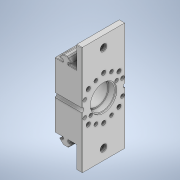
# Autodesk Inventor part: BearingMount
Saved by Autodesk Inventor 2020 (Build 240168000, 168)
## iProperties
Created: 2020-01-07
Part Number: BearingMount
Material: Generic
Document SubType Name: Modeling
Designer: srini
Density: 1 g/cm^3
Appearance: Default
Author: srini
Autodesk Inventor part; units mm, degrees
ref_plane "YZ Plane" through (0, 0, 0) normal (1, 0, 0) x (0, 1, 0)
ref_plane "XZ Plane" through (0, 0, 0) normal (0, 1, 0) x (-1, 0, 0)
ref_plane "XY Plane" through (0, 0, 0) normal (0, 0, 1) x (1, 0, 0)
sketch "Sketch1" plane through (0, 0, 0) normal (0, 0, 1) x (1, 0, 0)
  arc A0 (3.4842, -10.3402) -> (2.8892, -12.7) centre (3.4842, -11.5951) ccw construction
  line L0 (3.4842, -10.3402) -> (5.6567, -10.3402) construction
  arc A1 (5.6567, -10.3402) -> (6.269, -8.8618) centre (5.6567, -9.4742) ccw construction
  line L1 (6.269, -8.8618) -> (2.9517, -5.5445) construction
  line L2 (0.8127, -4.6585) -> (-2.4489, -4.6585) construction
  arc A2 (2.9517, -5.5445) -> (0.8127, -4.6585) centre (0.8127, -7.6835) ccw construction
  arc A3 (-2.4489, -4.6585) -> (-4.5879, -5.5445) centre (-2.4489, -7.6835) ccw construction
  line L3 (-4.5879, -5.5445) -> (-7.9053, -8.8618) construction
  arc A4 (-7.9053, -8.8618) -> (-7.2929, -10.3402) centre (-7.2929, -9.4742) ccw construction
  line L4 (-7.2929, -10.3402) -> (-5.1204, -10.3402) construction
  arc A5 (-4.5255, -12.7) -> (-5.1204, -10.3402) centre (-5.1204, -11.5951) ccw construction
  arc A6 (2.8892, -88.9) -> (3.4842, -91.2598) centre (3.4842, -90.0049) ccw construction
  line L5 (5.6567, -91.2598) -> (3.4842, -91.2598) construction
  arc A7 (6.269, -92.7382) -> (5.6567, -91.2598) centre (5.6567, -92.1258) ccw construction
  line L6 (2.9517, -96.0555) -> (6.269, -92.7382) construction
  arc A8 (0.8127, -96.9415) -> (2.9517, -96.0555) centre (0.8127, -93.9165) ccw construction
  line L7 (-2.4489, -96.9415) -> (0.8127, -96.9415) construction
  arc A9 (-4.5879, -96.0555) -> (-2.4489, -96.9415) centre (-2.4489, -93.9165) ccw construction
  line L8 (-7.9053, -92.7382) -> (-4.5879, -96.0555) construction
  arc A10 (-7.2929, -91.2598) -> (-7.9053, -92.7382) centre (-7.2929, -92.1258) ccw construction
  line L9 (-5.1204, -91.2598) -> (-7.2929, -91.2598) construction
  arc A11 (-5.1204, -91.2598) -> (-4.5255, -88.9) centre (-5.1204, -90.0049) ccw construction
  line L10 (18.2319, -12.7) -> (2.8892, -12.7)
  line L11 (-13.5181, -12.7) -> (-13.5181, -88.9)
  line L12 (-13.5181, -88.9) -> (-4.5255, -88.9)
  line L13 (18.2319, -88.9) -> (18.2319, -12.7)
  line L14 (-13.5181, -6.3246) -> (-13.5181, -9.5504) projected
  line L15 (2.8892, -12.7) -> (2.4625, -12.7)
  line L16 (-4.5255, -12.7) -> (-13.5181, -12.7)
  line L17 (2.8892, -88.9) -> (18.2319, -88.9)
  line L18 (-4.5255, -88.9) -> (-4.0987, -88.9)
  line L19 (18.2319, 12.7) -> (11.8819, 12.7)
  line L20 (11.8819, 12.7) -> (11.8819, -114.3)
  line L21 (11.8819, -114.3) -> (18.2319, -114.3)
  line L22 (18.2319, -114.3) -> (18.2319, 12.7)
  line L23 (8.7323, 12.7) -> (5.5065, 12.7) projected
  arc A12 (2.4625, -88.9) -> (3.4842, -91.5098) centre (3.4842, -90.0049) ccw
  line L24 (3.4842, -91.5098) -> (5.6567, -91.5098)
  arc A13 (6.0922, -92.5614) -> (5.6567, -91.5098) centre (5.6567, -92.1258) ccw
  line L25 (6.0922, -92.5614) -> (2.7749, -95.8787)
  arc A14 (0.8127, -96.6915) -> (2.7749, -95.8787) centre (0.8127, -93.9165) ccw
  line L26 (0.8127, -96.6915) -> (-2.4489, -96.6915)
  arc A15 (-4.4112, -95.8787) -> (-2.4489, -96.6915) centre (-2.4489, -93.9165) ccw
  line L27 (-4.4112, -95.8787) -> (-7.7285, -92.5614)
  arc A16 (-7.2929, -91.5098) -> (-7.7285, -92.5614) centre (-7.2929, -92.1258) ccw
  line L28 (-7.2929, -91.5098) -> (-5.1204, -91.5098)
  arc A17 (-5.1204, -91.5098) -> (-4.0987, -88.9) centre (-5.1204, -90.0049) ccw
  line L29 (-4.0987, -88.9) -> (2.4625, -88.9)
  line L30 (2.4625, -88.9) -> (2.8892, -88.9)
  arc A18 (-4.0987, -12.7) -> (-5.1204, -10.0902) centre (-5.1204, -11.5951) ccw
  line L31 (-5.1204, -10.0902) -> (-7.2929, -10.0902)
  arc A19 (-7.7285, -9.0386) -> (-7.2929, -10.0902) centre (-7.2929, -9.4742) ccw
  line L32 (-7.7285, -9.0386) -> (-4.4112, -5.7213)
  arc A20 (-2.4489, -4.9085) -> (-4.4112, -5.7213) centre (-2.4489, -7.6835) ccw
  line L33 (-2.4489, -4.9085) -> (0.8127, -4.9085)
  arc A21 (2.7749, -5.7213) -> (0.8127, -4.9085) centre (0.8127, -7.6835) ccw
  line L34 (2.7749, -5.7213) -> (6.0922, -9.0386)
  arc A22 (5.6567, -10.0902) -> (6.0922, -9.0386) centre (5.6567, -9.4742) ccw
  line L35 (5.6567, -10.0902) -> (3.4842, -10.0902)
  arc A23 (3.4842, -10.0902) -> (2.4625, -12.7) centre (3.4842, -11.5951) ccw
  line L36 (-4.0987, -12.7) -> (-4.5255, -12.7)
  line L37 (2.4625, -12.7) -> (-4.0987, -12.7)
  point P0 (0, 0)
  point P1 (11.8819, -12.7)
  point P2 (11.8819, -88.9)
  dimension "d0" = 31.75
  dimension "d1" = 127
  dimension "d2" = 6.35
  dimension "d81" = 0.25
  dimension "d82" = 0.25
  constraints: 52 end point, 28 parallel, 28 point on circle, 12 centre point, 6 horizontal, 6 perpendicular, 3 collinear, 1 point on line, 20 other
  measures "d0" distance of L10.start L11.start
  measures "d1" distance of L21.end L19.start
  measures "d2" distance of L19.start L19.end
  measures "d81" distance between parallel lines of L26 L7
  measures "d82" distance between parallel lines of L2 L33
extrude "Extrusion1" add sketch "Sketch1" along normal blind 50.8
sketch "Sketch2" plane through (18.2319, -114.3, 0) normal (1, 0, 0) x (0, 0, -1)
  circle A0 centre (-12.7, 114.3) radius 3.3734
  line L0 (0, 127) -> (-50.8, 127) projected
  line L1 (0, 0) -> (0, 127) projected
  circle A1 centre (-12.7, 12.7) radius 3.3734
  circle A2 centre (-25.4, 114.3) radius 3.3734
  circle A3 centre (-25.4, 12.7) radius 3.3734
  circle A4 centre (-25.4, 63.5) radius 12.9921
  circle A5 centre (-38.1, 114.3) radius 3.3734
  circle A6 centre (-38.1, 12.7) radius 3.3734
  point P0 (0, 114.3)
  dimension "d5" = 12.7
  dimension "d6" = 12.7
  dimension "d7" = 6.7469
  dimension "d10" = 101.6
  dimension "d13" = 12.7
  dimension "d29" = 63.5
  dimension "d30" = 25.4
  dimension "d31" = 25.9842
  constraints: 7 centre point, 1 horizontal, 1 vertical, 10 other
  measures "d5" distance from line of A0.centre L0
  measures "d6" distance from line of A0.centre L1
  measures "d7" diameter of A0
  measures "d10" distance of A0.centre A1.centre
  measures "d13" distance of A0.centre A2.centre
  measures "d29" distance from line of A4.centre L0
  measures "d30" distance from line of A4.centre L1
  measures "d31" diameter of A4
extrude "Extrusion2" cut sketch "Sketch2" against normal through all contours A2 | A3 | A4
sketch "Sketch4" plane through (18.2319, -114.3, 0) normal (1, 0, 0) x (0, 0, -1)
  circle A0 centre (-25.4, 63.5) radius 12.9921 projected
  circle A1 centre (-25.4, 63.5) radius 14.3002
  point P0 (0, 114.3)
  dimension "d32" = 28.6004
  constraints: 1 centre point, 1 coincident
  measures "d32" diameter of A1
extrude "Extrusion4" cut sketch "Sketch4" against normal blind 7.9756 contours A0 | A1
sketch "Sketch5" plane through (18.2319, -114.3, 0) normal (1, 0, 0) x (0, 0, -1)
  circle A0 centre (-25.4, 63.5) radius 14.3002 projected
  circle A1 centre (-25.4, 63.5) radius 15.5702
  point P0 (0, 114.3)
  dimension "d35" = 31.1404
  constraints: 1 centre point, 1 coincident
  measures "d35" diameter of A1
extrude "Extrusion5" cut sketch "Sketch5" against normal blind 1.6256 contours A0 | A1
sketch "Sketch6" plane through (-13.5181, -88.9, 0) normal (-1, 0, 0) x (0, 0, 1)
  circle A0 centre (25.4, 38.1) radius 12.9921 projected
  circle A1 centre (25.4, 38.1) radius 14.3002
  point P0 (0, 88.9)
  dimension "d41" = 28.6004
  constraints: 1 centre point, 1 coincident
  measures "d41" diameter of A1
extrude "Extrusion6" cut sketch "Sketch6" against normal blind 7.9756 contours A0 | A1
sketch "Sketch7" plane through (-13.5181, -88.9, 0) normal (-1, 0, 0) x (0, 0, 1)
  circle A0 centre (25.4, 38.1) radius 14.3002 projected
  circle A1 centre (25.4, 38.1) radius 15.5702
  point P0 (0, 88.9)
  dimension "d44" = 31.1404
  constraints: 1 centre point, 1 coincident
  measures "d44" diameter of A1
extrude "Extrusion7" cut sketch "Sketch7" against normal blind 1.6256 contours A0 | A1
sketch "Sketch8" plane through (-13.5181, -88.9, 0) normal (-1, 0, 0) x (0, 0, 1)
  circle A0 centre (10.3089, 48.1835) radius 2.0955
  circle A1 centre (40.4911, 28.0165) radius 2.0955
  line L0 (10.3089, 48.1835) -> (40.4911, 28.0165)
  circle A2 centre (25.4, 38.1) radius 12.9921 projected
  line L1 (50.8, -25.4) -> (50.8, 101.6) projected
  point P0 (0, 88.9)
  dimension "d50" = 36.2998
  dimension "d51" = 4.191
  dimension "d74" = 56.25
  constraints: 2 centre point, 2 end point, 1 coincident, 1 equal radius, 1 midpoint
  measures "d50" distance of L0.start L0.end
  measures "d51" diameter of A0
  measures "d74" angle of L0 L1
extrude "Extrusion8" cut sketch "Sketch8" against normal through all contours A0 | A1
chamfer "Chamfer3" distance 0.635 angle 45 18 edges at (11.8819, 0, 50.8) (-13.5181, -50.8, 50.8) (15.0569, 12.7, 50.8) (18.2319, -50.8, 50.8) (11.8819, -101.6, 50.8) (15.0569, -114.3, 50.8) (15.0569, -114.3, 0) (11.8819, -101.6, 0) (-13.5181, -50.8, 0) (18.2319, -50.8, 0) (11.8819, 0, 0) (15.0569, 12.7, 0) (11.8819, -101.6, 28.7734) (18.2319, -101.6, 28.7734) (18.2319, 0, 28.7734) (11.8819, 0, 28.7734) (-13.5181, -12.7, 25.4) (-13.5181, -88.9, 25.4)
sketch "Sketch9" plane through (18.2319, -114.3, 0.635) normal (1, 0, 0) x (0, 0, -1)
  circle A0 centre (-24.765, 38.1) radius 2.4892
  circle A1 centre (-24.765, 63.5) radius 12.9921 projected
  circle A2 centre (-6.8045, 45.5395) radius 2.4892
  circle A3 centre (0.635, 63.5) radius 2.4892
  circle A4 centre (-6.8045, 81.4605) radius 2.4892
  circle A5 centre (-24.765, 88.9) radius 2.4892
  circle A6 centre (-42.7255, 81.4605) radius 2.4892
  circle A7 centre (-50.165, 63.5) radius 2.4892
  circle A8 centre (-42.7255, 45.5395) radius 2.4892
  point P0 (0.635, 114.3)
  dimension "d57" = 25.4
  dimension "d58" = 4.9784
  dimension "d61" = 360
  constraints: 8 centre point, 1 vertical alignment, 17 other
  measures "d57" distance of A1.centre A0.centre
  measures "d58" diameter of A0
extrude "Extrusion9" cut sketch "Sketch9" against normal through all contours A0 | A2 | A3 | A4 | A5 | A6 | A7 | A8
sketch "Sketch10" plane through (-13.5181, -88.9, 0.635) normal (-1, 0, 0) x (0, 0, 1)
  circle A0 centre (15.6524, 16.1001) radius 2.1526
  circle A1 centre (24.765, 38.1) radius 12.9921 construction
  circle A2 centre (24.765, 12.7) radius 2.4892 projected
  line L0 (24.765, 12.7) -> (24.765, 38.1) construction
  line L1 (24.765, 38.1) -> (15.6524, 16.1001) construction
  line L2 (24.765, 38.1) -> (33.8776, 16.1001) construction
  circle A3 centre (33.8776, 16.1001) radius 2.1526
  line L3 (24.765, 38.1) -> (46.7649, 28.9874) construction
  circle A4 centre (46.7649, 28.9874) radius 2.1526
  line L4 (24.765, 38.1) -> (46.7649, 47.2126) construction
  circle A5 centre (46.7649, 47.2126) radius 2.1526
  line L5 (24.765, 38.1) -> (33.8776, 60.0999) construction
  circle A6 centre (33.8776, 60.0999) radius 2.1526
  line L6 (24.765, 38.1) -> (15.6524, 60.0999) construction
  circle A7 centre (15.6524, 60.0999) radius 2.1526
  line L7 (24.765, 38.1) -> (2.7651, 47.2126) construction
  circle A8 centre (2.7651, 47.2126) radius 2.1526
  line L8 (24.765, 38.1) -> (2.7651, 28.9874) construction
  circle A9 centre (2.7651, 28.9874) radius 2.1526
  point P0 (-0.635, 88.9)
  dimension "d65" = 4.3053
  dimension "d66" = 23.8125
  dimension "d67" = 22.5
  dimension "d70" = 360
  constraints: 18 end point, 8 centre point, 2 coincident, 1 vertical, 31 other
  measures "d65" diameter of A0
  measures "d66" distance of L0.end L1.end
  measures "d67" angle of L1 L0
extrude "Extrusion10" cut sketch "Sketch10" against normal through all contours A0 | A3 | A4 | A5 | A6 | A7 | A8 | A9
sketch "Sketch11" plane through (11.8819, -12.7, 0.635) normal (-1, 0, 0) x (0, 0, 1)
  line L0 (28.1384, 9.3266) -> (21.3916, 9.3266)
  line L1 (21.3916, 9.3266) -> (21.3916, 16.0734)
  line L2 (21.3916, 16.0734) -> (28.1384, 16.0734)
  line L3 (28.1384, 16.0734) -> (28.1384, 9.3266)
  circle A0 centre (24.765, 12.7) radius 3.3734 projected
  line L4 (28.1384, 9.3266) -> (21.3916, 16.0734) construction
  line L5 (21.3916, 9.3266) -> (28.1384, 16.0734) construction
  line L6 (28.1384, -85.5266) -> (21.3916, -85.5266)
  line L7 (21.3916, -85.5266) -> (21.3916, -92.2734)
  line L8 (21.3916, -92.2734) -> (28.1384, -92.2734)
  line L9 (28.1384, -92.2734) -> (28.1384, -85.5266)
  circle A1 centre (24.765, -88.9) radius 3.3734 projected
  line L10 (28.1384, -85.5266) -> (21.3916, -92.2734) construction
  line L11 (21.3916, -85.5266) -> (28.1384, -92.2734) construction
  point P0 (-0.635, 12.7)
  constraints: 24 end point, 4 midpoint, 4 parallel, 4 tangent, 2 horizontal, 2 perpendicular
extrude "Extrusion11" cut sketch "Sketch11" against normal blind 3.175
sketch "Sketch12" plane through (11.8819, -114.3, 0.635) normal (-1, 0, 0) x (0, 0, 1)
  circle A0 centre (24.765, 12.7) radius 3.3734 projected
  circle A1 centre (24.765, 12.7) radius 7.62
  circle A2 centre (24.765, 114.3) radius 3.3734 projected
  circle A3 centre (24.765, 114.3) radius 7.62
  point P0 (-0.635, 114.3)
  dimension "d77" = 15.24
  dimension "d78" = 15.24
  constraints: 2 centre point, 2 coincident
  measures "d77" diameter of A1
  measures "d78" diameter of A3
extrude "Extrusion12" cut sketch "Sketch12" along normal through all contours A0 | A1 | A2 | A3
fillet "Fillet1" radius 0.635 4 edges at (-4.0987, -12.7, 25.4) (2.4625, -12.7, 25.4) (-4.0987, -88.9, 25.4) (2.4625, -88.9, 25.4)
chamfer "Chamfer4" distance 0.508 angle 45 60 edges at (-3.7998, -10.8735, 0) (-4.0839, -12.6222, 0) (-8.6358, -12.7, 0) (-6.2067, -10.0902, 0) (-7.862, -9.7099, 0) (-6.0698, -7.38, 0) (-3.5109, -5.1197, 0) (-0.8181, -4.9085, 0) (1.8746, -5.1197, 0) (4.4336, -7.38, 0) (6.2258, -9.7099, 0) (4.5704, -10.0902, 0) (2.1636, -10.8735, 0) (2.4476, -12.6222, 0) (7.6345, -12.7, 0) (-8.6358, -12.7, 50.8) (-4.0839, -12.6222, 50.8) (-3.7998, -10.8735, 50.8) (-6.2067, -10.0902, 50.8) (-7.862, -9.7099, 50.8) (-6.0698, -7.38, 50.8) (-3.5109, -5.1197, 50.8) (-0.8181, -4.9085, 50.8) (1.8746, -5.1197, 50.8) (4.4336, -7.38, 50.8) (6.2258, -9.7099, 50.8) (4.5704, -10.0902, 50.8) (2.1636, -10.8735, 50.8) (2.4476, -12.6222, 50.8) (7.6345, -12.7, 50.8) (-8.6358, -88.9, 50.8) (-4.0839, -88.9778, 50.8) (-3.7998, -90.7265, 50.8) (-6.2067, -91.5098, 50.8) (-7.862, -91.8901, 50.8) (-6.0698, -94.22, 50.8) (-3.5109, -96.4803, 50.8) (-0.8181, -96.6915, 50.8) (1.8746, -96.4803, 50.8) (4.4336, -94.22, 50.8) (6.2258, -91.8901, 50.8) (4.5704, -91.5098, 50.8) (2.1636, -90.7265, 50.8) (2.4476, -88.9778, 50.8) (7.6345, -88.9, 50.8) (-8.6358, -88.9, 0) (-4.0839, -88.9778, 0) (-3.7998, -90.7265, 0) (-6.2067, -91.5098, 0) (-7.862, -91.8901, 0) (-6.0698, -94.22, 0) (-3.5109, -96.4803, 0) (-0.8181, -96.6915, 0) (1.8746, -96.4803, 0) (4.4336, -94.22, 0) (6.2258, -91.8901, 0) (4.5704, -91.5098, 0) (2.1636, -90.7265, 0) (2.4476, -88.9778, 0) (7.6345, -88.9, 0)
equation "\"d82\" = d81"
body "Solid1"
